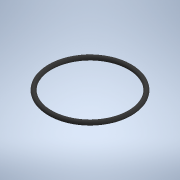
# Autodesk Inventor part: Oring 2-026
Saved by Autodesk Inventor 2020 (Build 240168000, 168)
## iProperties
Created: 2020-06-24
Part Number: Oring 2-026
Material: Rubber
Document SubType Name: Modeling
Designer: Juan
Density: 0.93 g/cm^3
Appearance: Rubber - Black
Author: Juan
Autodesk Inventor part; units mm, degrees
ref_plane "YZ Plane" through (0, 0, 0) normal (1, 0, 0) x (0, 1, 0)
ref_plane "XZ Plane" through (0, 0, 0) normal (0, 1, 0) x (-1, 0, 0)
ref_plane "XY Plane" through (0, 0, 0) normal (0, 0, 1) x (1, 0, 0)
sketch "Sketch1" plane through (0, 0, 0) normal (1, 0, 0) x (0, 1, 0)
  circle A0 centre (0, 16.625) radius 0.89
  line L0 (0, 0) -> (2.0755, 0)
  dimension "d0" = 1.78
  dimension "d1" = 16.625
  constraints: 2 end point, 1 centre point, 1 horizontal
  measures "d0" diameter of A0
  measures "d1" distance of L0.start A0.centre
revolve "Revolution1" add sketch "Sketch1" angle 360 about axis through (0, 0, 0) along (0, 1, 0)
body "Solid1"
